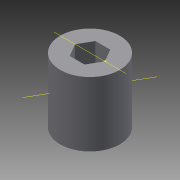
# Autodesk Inventor part: bics-eng-base
Saved by Autodesk Inventor 2015 SP1 (Build 190203100, 203)
## iProperties
Created: 2015-06-17
Part Number: bics-eng-base
Material: Genérico
Document SubType Name: Modeling
Designer: Javier
Density: 1 g/cm^3
Appearance: Valor por defecto
Author: Javier
Autodesk Inventor part; units mm, degrees
ref_plane "YZ Plane" through (0, 0, 0) normal (1, 0, 0) x (0, 1, 0)
ref_plane "XZ Plane" through (0, 0, 0) normal (0, 1, 0) x (-1, 0, 0)
ref_plane "XY Plane" through (0, 0, 0) normal (0, 0, 1) x (1, 0, 0)
sketch "Boceto1" plane through (0, 0, 0) normal (0, 0, 1) x (1, 0, 0)
  line L0 (4, 0) -> (2, -3.4641)
  line L1 (2, -3.4641) -> (-2, -3.4641)
  line L2 (-2, -3.4641) -> (-4, 0)
  line L3 (-4, 0) -> (-2, 3.4641)
  line L4 (-2, 3.4641) -> (2, 3.4641)
  line L5 (2, 3.4641) -> (4, 0)
  circle A0 centre (0, 0) radius 6
  dimension "d0" = 8
  dimension "d1" = 12
  constraints: 12 end point, 2 coincident, 1 centre point, 13 other
  measures "d0" distance of L0.start L2.end
  measures "d1" diameter of A0
extrude "Extrusión1" add sketch "Boceto1" along normal blind 7
sketch "Boceto2" plane through (0, 0, 7) normal (0, 0, 1) x (1, 0, 0)
  line L0 (3, 0) -> (1.5, -2.5981)
  line L1 (1.5, -2.5981) -> (-1.5, -2.5981)
  line L2 (-1.5, -2.5981) -> (-3, 0)
  line L3 (-3, 0) -> (-1.5, 2.5981)
  line L4 (-1.5, 2.5981) -> (1.5, 2.5981)
  line L5 (1.5, 2.5981) -> (3, 0)
  circle A0 centre (0, 0) radius 6 projected
  constraints: 12 end point, 1 coincident, 13 other
extrude "Extrusión2" add sketch "Boceto2" along normal blind 6
